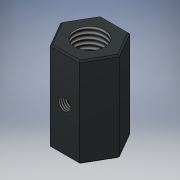
# Autodesk Inventor part: КВ33.000.105 - Каретка
Saved by Autodesk Inventor 2019 (Build 230136000, 136)
## iProperties
Created: 2021-04-18
Part Number: КВ33.000.105 - Каретка
Material: Iron, Cast
Document SubType Name: Modeling
Designer: Петров Иван
Density: 7.15 g/cm^3
Appearance: Iron Gray
Author: Петров Иван
Autodesk Inventor part; units mm, degrees
ref_plane "YZ Plane" through (0, 0, 0) normal (1, 0, 0) x (0, 1, 0)
ref_plane "XZ Plane" through (0, 0, 0) normal (0, 1, 0) x (-1, 0, 0)
ref_plane "XY Plane" through (0, 0, 0) normal (0, 0, 1) x (1, 0, 0)
sketch "Sketch1" plane through (0, 0, 0) normal (0, 1, 0) x (-1, 0, 0)
  circle A0 centre (0, 0) radius 5
  line L0 (9.815, 0) -> (4.9075, -8.5)
  line L1 (4.9075, -8.5) -> (-4.9075, -8.5)
  line L2 (-4.9075, -8.5) -> (-9.815, 0)
  line L3 (-9.815, 0) -> (-4.9075, 8.5)
  line L4 (-4.9075, 8.5) -> (4.9075, 8.5)
  line L5 (4.9075, 8.5) -> (9.815, 0)
  dimension "d0" = 10
  dimension "d1" = 17
  constraints: 12 end point, 2 coincident, 1 centre point, 13 other
  measures "d0" diameter of A0
  measures "d1" distance between parallel lines of L1 L4
extrude "Extrusion1" add sketch "Sketch1" along normal blind 30
chamfer "Chamfer1" distance 0.5 angle 45 12 edges at (7.3612, 0, 4.25) (0, 0, 8.5) (-7.3612, 0, 4.25) (-7.3612, 0, -4.25) (0, 0, -8.5) (7.3612, 0, -4.25) (7.3612, 30, -4.25) (7.3612, 30, 4.25) (0, 30, 8.5) (-7.3612, 30, 4.25) (-7.3612, 30, -4.25) (0, 30, -8.5)
thread "Thread1" size "M10x1.5" class "6H" standard "ANSI Metric M Profile" full length
sketch "Sketch2" plane through (-4.9075, 29.5, 8.5) normal (0, 0, 1) x (1, 0, 0)
  circle A0 centre (4.9075, -14.5) radius 2
  point P0 (4.9075, -29.5)
  dimension "d9" = 4
  dimension "d10" = 15
  constraints: 1 centre point, 1 vertical alignment
  measures "d9" diameter of A0
  measures "d10" distance of point (4.907, -29.5) A0.centre
extrude "Extrusion2" cut sketch "Sketch2" against normal blind 26.75
thread "Thread2" size "M4x0.7" class "6H" standard "ANSI Metric M Profile" full length
thread "Thread3" size "M4x0.7" class "6H" standard "ANSI Metric M Profile" full length
body "Solid1"
